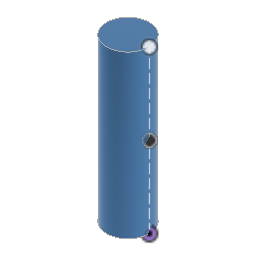
2200mAh Battery Holder (Autodesk Fusion 360 archive; units mm, degrees)
design "LiPo_Bat_2200_Single_Cell"
Autodesk Fusion 360 part; units mm, degrees
sketch "Sketch1" plane through (0, 0, 0) normal (0, 0, 1) x (1, 0, 0)
  circle A0 centre (0, 0) radius 9.25
  dimension "d1" = 18.5
  constraint coincident A0.centre origin
  measures "d1" diameter of A0
extrude "Extrude1" add sketch "Sketch1" along normal blind 70
ref_plane "WorkPlane1" through (9.25, 0, 0) normal (1, 0, 0) x (0, 1, 0)
sketch "Sketch2" plane through (9.25, 0, 0) normal (1, 0, 0) x (0, 1, 0)
  line L0 (0, 0) -> (0, 70) construction
  point P0 (0, 35)
  constraint coincident L0.start origin
  constraint vertical L0
  constraint midpoint L0 P0
equation "d8 = ( 18.5 / 2 ) * 1 mm"
